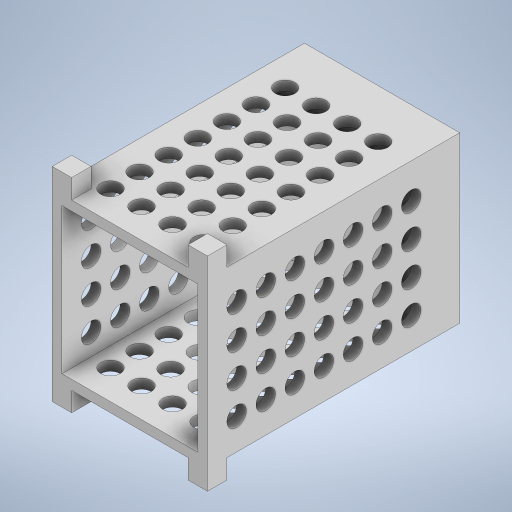
# Autodesk Inventor part: battery_box_ver2
Saved by Autodesk Inventor 2023 (Build 270158000, 158)
## iProperties
Created: 2023-05-21
Part Number: battery_box_ver2
Material: 一般
Document SubType Name: Modeling
Designer: 310611102
Density: 1 g/cm^3
Appearance: 預設
Author: 310611102
Autodesk Inventor part; units mm, degrees
ref_plane "YZ Plane" through (0, 0, 0) normal (1, 0, 0) x (0, 1, 0)
ref_plane "XZ Plane" through (0, 0, 0) normal (0, 1, 0) x (-1, 0, 0)
ref_plane "XY Plane" through (0, 0, 0) normal (0, 0, 1) x (1, 0, 0)
sketch "Sketch1" plane through (0, 0, 0) normal (0, 0, 1) x (1, 0, 0)
  line L0 (-40, 42.5) -> (40, 42.5)
  line L1 (40, 42.5) -> (40, -42.5)
  line L2 (40, -42.5) -> (-40, -42.5)
  line L3 (-40, -42.5) -> (-40, 42.5)
  line L4 (-40, 42.5) -> (40, -42.5) construction
  line L5 (40, 42.5) -> (-40, -42.5) construction
  point P0 (0, 0)
  dimension "d0" = 85
  dimension "d1" = 80
  constraints: 12 end point, 2 midpoint, 2 parallel, 1 horizontal, 1 perpendicular
  measures "d0" distance of L0.end L1.end
  measures "d1" distance of L0.start L0.end
extrude "Extrusion1" add sketch "Sketch1" along normal blind 20
sketch "Sketch2" plane through (0, 0, 20) normal (0, 0, 1) x (1, 0, 0)
  line L0 (-35, 37.5) -> (35, 37.5)
  line L1 (35, 37.5) -> (35, -37.5)
  line L2 (35, -37.5) -> (-35, -37.5)
  line L3 (-35, -37.5) -> (-35, 37.5)
  line L4 (-35, 37.5) -> (35, -37.5) construction
  line L5 (35, 37.5) -> (-35, -37.5) construction
  line L6 (40, -42.5) -> (40, 42.5)
  line L7 (40, 42.5) -> (-40, 42.5)
  line L8 (-40, 42.5) -> (-40, -42.5)
  line L9 (-40, -42.5) -> (40, -42.5)
  point P0 (0, 0)
  dimension "d4" = 75
  dimension "d5" = 70
  dimension "d6" = 5
  constraints: 20 end point, 4 parallel, 2 midpoint, 2 perpendicular, 1 horizontal, 3 other
  measures "d4" distance of L0.end L1.end
  measures "d5" distance of L0.start L0.end
  measures "d6" distance between parallel lines of L1 L6
extrude "Extrusion2" add sketch "Sketch2" along normal blind 110
sketch "Sketch3" plane through (0, 0, 0) normal (0, 0, -1) x (-1, 0, 0)
  circle A0 centre (-35, 37.5) radius 2.5
  line L0 (-40, 42.5) -> (40, 42.5) projected
  line L1 (-40, -42.5) -> (-40, 42.5) projected
  line L2 (-35, 37.5) -> (-25.2876, 37.5)
  line L3 (-25.2876, 37.5) -> (-25.2876, 30.7478)
  circle A1 centre (35, 37.5) radius 2.5
  circle A2 centre (-35, -37.5) radius 2.5
  circle A3 centre (35, -37.5) radius 2.5
  point P0 (0, 0)
  dimension "d9" = 5
  dimension "d10" = 5
  dimension "d11" = 5
  dimension "d14" = 70
  dimension "d17" = 75
  constraints: 4 centre point, 4 end point, 2 horizontal, 1 perpendicular, 1 vertical, 6 other
  measures "d9" diameter of A0
  measures "d10" distance from line of L0 L2.start
  measures "d11" distance from line of L1 L2.start
  measures "d14" distance of L2.start A1.centre
  measures "d17" distance of L2.start A2.centre
extrude "Extrusion3" cut sketch "Sketch3" against normal blind 10
sketch "Sketch4" plane through (-40, -42.5, 0) normal (0, -1, 0) x (1, 0, 0)
  line L0 (0, 130) -> (80, 130) projected
  line L1 (0, 0) -> (0, 130) projected
  circle A0 centre (15, 115) radius 5
  circle A1 centre (31, 115) radius 5
  circle A2 centre (47, 115) radius 5
  circle A3 centre (63, 115) radius 5
  circle A4 centre (15, 100) radius 5
  circle A5 centre (31, 100) radius 5
  circle A6 centre (47, 100) radius 5
  circle A7 centre (63, 100) radius 5
  circle A8 centre (15, 85) radius 5
  circle A9 centre (31, 85) radius 5
  circle A10 centre (47, 85) radius 5
  circle A11 centre (63, 85) radius 5
  circle A12 centre (15, 70) radius 5
  circle A13 centre (31, 70) radius 5
  circle A14 centre (47, 70) radius 5
  circle A15 centre (63, 70) radius 5
  circle A16 centre (15, 55) radius 5
  circle A17 centre (31, 55) radius 5
  circle A18 centre (47, 55) radius 5
  circle A19 centre (63, 55) radius 5
  circle A20 centre (15, 40) radius 5
  circle A21 centre (31, 40) radius 5
  circle A22 centre (47, 40) radius 5
  circle A23 centre (63, 40) radius 5
  circle A24 centre (15, 25) radius 5
  circle A25 centre (31, 25) radius 5
  circle A26 centre (47, 25) radius 5
  circle A27 centre (63, 25) radius 5
  point P0 (40, 0)
  dimension "d27" = 10
  dimension "d28" = 15
  dimension "d29" = 15
  dimension "d32" = 16
  dimension "d35" = 15
  constraints: 28 centre point, 1 horizontal, 1 vertical, 54 other
  measures "d27" diameter of A0
  measures "d28" distance from line of L0 A0.centre
  measures "d29" distance from line of L1 A0.centre
  measures "d32" distance of A0.centre A1.centre
  measures "d35" distance of A0.centre A4.centre
extrude "Extrusion4" cut sketch "Sketch4" against normal through all
sketch "Sketch5" plane through (40, -42.5, 0) normal (1, 0, 0) x (0, 0, -1)
  circle A0 centre (-115, 16) radius 5
  line L0 (-130, 0) -> (-130, 85) projected
  line L1 (0, 0) -> (-130, 0) projected
  circle A1 centre (-115, 33) radius 5
  circle A2 centre (-115, 50) radius 5
  circle A3 centre (-115, 67) radius 5
  circle A4 centre (-100, 16) radius 5
  circle A5 centre (-100, 33) radius 5
  circle A6 centre (-100, 50) radius 5
  circle A7 centre (-100, 67) radius 5
  circle A8 centre (-85, 16) radius 5
  circle A9 centre (-85, 33) radius 5
  circle A10 centre (-85, 50) radius 5
  circle A11 centre (-85, 67) radius 5
  circle A12 centre (-70, 16) radius 5
  circle A13 centre (-70, 33) radius 5
  circle A14 centre (-70, 50) radius 5
  circle A15 centre (-70, 67) radius 5
  circle A16 centre (-55, 16) radius 5
  circle A17 centre (-55, 33) radius 5
  circle A18 centre (-55, 50) radius 5
  circle A19 centre (-55, 67) radius 5
  circle A20 centre (-40, 16) radius 5
  circle A21 centre (-40, 33) radius 5
  circle A22 centre (-40, 50) radius 5
  circle A23 centre (-40, 67) radius 5
  circle A24 centre (-25, 16) radius 5
  circle A25 centre (-25, 33) radius 5
  circle A26 centre (-25, 50) radius 5
  circle A27 centre (-25, 67) radius 5
  point P0 (0, 42.5)
  dimension "d40" = 10
  dimension "d41" = 15
  dimension "d42" = 16
  dimension "d45" = 17
  dimension "d48" = 15
  constraints: 28 centre point, 1 horizontal, 1 vertical, 54 other
  measures "d40" diameter of A0
  measures "d41" distance from line of L0 A0.centre
  measures "d42" distance from line of L1 A0.centre
  measures "d45" distance of A0.centre A1.centre
  measures "d48" distance of A0.centre A4.centre
extrude "Extrusion5" cut sketch "Sketch5" against normal through all
sketch "Sketch6" plane through (0, 0, 130) normal (0, 0, 1) x (1, 0, 0)
  line L0 (-40, 42.5) -> (-30, 42.5)
  line L1 (-30, 42.5) -> (-30, 52.5)
  line L2 (-30, 52.5) -> (-40, 52.5)
  line L3 (-40, 52.5) -> (-40, 42.5)
  line L4 (40, -42.5) -> (40, 42.5) projected
  line L5 (40, 42.5) -> (30, 42.5)
  line L6 (30, 42.5) -> (30, 52.5)
  line L7 (30, 52.5) -> (40, 52.5)
  line L8 (40, 52.5) -> (40, 42.5)
  line L9 (40, -42.5) -> (30, -42.5)
  line L10 (30, -42.5) -> (30, -52.5)
  line L11 (30, -52.5) -> (40, -52.5)
  line L12 (40, -52.5) -> (40, -42.5)
  line L13 (-40, -42.5) -> (40, -42.5) projected
  line L14 (-40, -42.5) -> (-30, -42.5)
  line L15 (-30, -42.5) -> (-30, -52.5)
  line L16 (-30, -52.5) -> (-40, -52.5)
  line L17 (-40, -52.5) -> (-40, -42.5)
  dimension "d59" = 10
  dimension "d60" = 10
  dimension "d61" = 10
  dimension "d62" = 10
  constraints: 32 end point, 8 parallel, 4 horizontal, 4 perpendicular, 3 collinear, 1 coincident, 1 point on line
  measures "d59" distance of L1.end L2.end
  measures "d60" distance of L2.end L0.start
  measures "d61" distance of L6.end L7.end
  measures "d62" distance of L11.end L4.start
extrude "Extrusion6" add sketch "Sketch6" against normal blind 10
body "Solid1"
